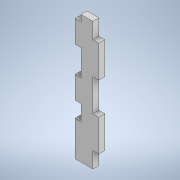
# Autodesk Inventor part: cover
Saved by Autodesk Inventor 2020 (Build 240168000, 168)
## iProperties
Created: 2019-12-19
Part Number: cover
Material: Générique
Document SubType Name: Modeling
Designer: damien
Density: 1 g/cm^3
Appearance: Par défaut
Author: damien
Autodesk Inventor part; units mm, degrees
ref_plane "YZ Plane" through (0, 0, 0) normal (1, 0, 0) x (0, 1, 0)
ref_plane "XZ Plane" through (0, 0, 0) normal (0, 1, 0) x (-1, 0, 0)
ref_plane "XY Plane" through (0, 0, 0) normal (0, 0, 1) x (1, 0, 0)
sketch "Esquisse3" plane through (0, 0, 0) normal (0, 0, 1) x (1, 0, 0)
  line L0 (37.1, -200) -> (-37.1, -200)
  line L1 (-37.1, -200) -> (-37.1, 200)
  line L2 (-37.1, 200) -> (37.1, 200)
  line L3 (37.1, 200) -> (37.1, -200)
  line L4 (37.1, -200) -> (-37.1, 200) construction
  line L5 (-37.1, -200) -> (37.1, 200) construction
  point P0 (0, 0)
  dimension "d20" = 74.2
  dimension "d21" = 400
  constraints: 12 end point, 2 midpoint, 2 parallel, 1 horizontal, 1 perpendicular
  measures "d20" distance of L0.start L0.end
  measures "d21" distance of L2.end L0.start
extrude "Extrusion3" add sketch "Esquisse3" along normal blind 18.55
sketch "Esquisse4" plane through (0, 0, 18.55) normal (0, 0, 1) x (1, 0, 0)
  line L0 (37.1, 200) -> (18.55, 200)
  line L1 (18.55, 200) -> (18.55, 150)
  line L2 (18.55, 150) -> (37.1, 150)
  line L3 (37.1, 150) -> (37.1, 200)
  line L4 (-37.1, -200) -> (37.1, -200) projected
  line L5 (37.1, -200) -> (18.55, -200)
  line L6 (18.55, -200) -> (18.55, -150)
  line L7 (18.55, -150) -> (37.1, -150)
  line L8 (37.1, -150) -> (37.1, -200)
  line L9 (37.1, -50) -> (18.55, -50)
  line L10 (18.55, -50) -> (18.55, 50)
  line L11 (18.55, 50) -> (37.1, 50)
  line L12 (37.1, 50) -> (37.1, -50)
  point P0 (0, 0)
  point P1 (18.55, -200)
  dimension "d24" = 50
  dimension "d25" = 50
  dimension "d27" = 100
  dimension "d29" = 100
  dimension "d30" = 100
  dimension "d31" = 18.55
  constraints: 24 end point, 6 parallel, 3 horizontal, 3 perpendicular, 2 collinear, 1 point on line
  measures "d24" distance of L5.end L6.end
  measures "d25" distance of L0.end L1.end
  measures "d27" distance of L9.end L10.end
  measures "d29" distance between parallel lines of L7 L9
  measures "d30" distance between parallel lines of L2 L11
  measures "d31" distance between parallel lines of L12 L10
extrude "Extrusion4" cut sketch "Esquisse4" against normal blind 18.55
sketch "Esquisse5" plane through (0, 0, 18.55) normal (0, 0, 1) x (1, 0, 0)
  line L0 (18.55, 200) -> (-37.1, 200) projected
  line L1 (-37.1, 200) -> (-18.55, 200)
  line L2 (-18.55, 200) -> (-18.55, 180)
  line L3 (-18.55, 180) -> (-37.1, 180)
  line L4 (-37.1, 180) -> (-37.1, 200)
  line L5 (-37.1, 200) -> (-37.1, -200) projected
  line L6 (-37.1, 110) -> (-18.55, 110)
  line L7 (-18.55, 110) -> (-18.55, 28.55)
  line L8 (-18.55, 28.55) -> (-37.1, 28.55)
  line L9 (-37.1, 28.55) -> (-37.1, 110)
  line L10 (-37.1, -41.45) -> (-18.55, -41.45)
  line L11 (-18.55, -41.45) -> (-18.55, -90.05)
  line L12 (-18.55, -90.05) -> (-37.1, -90.05)
  line L13 (-37.1, -90.05) -> (-37.1, -41.45)
  point P0 (0, 0)
  dimension "d34" = 20
  dimension "d35" = 18.55
  dimension "d37" = 70
  dimension "d38" = 81.45
  dimension "d39" = 70
  dimension "d40" = 48.6
  constraints: 24 end point, 6 parallel, 3 horizontal, 3 perpendicular, 2 collinear, 2 point on line
  measures "d34" distance of L3.end L0.end
  measures "d35" distance from line of L2 L3.end
  measures "d37" distance between parallel lines of L6 L3
  measures "d38" distance of L6.end L7.end
  measures "d39" distance between parallel lines of L10 L8
  measures "d40" distance of L10.end L11.end
extrude "Extrusion5" cut sketch "Esquisse5" against normal blind 18.55
